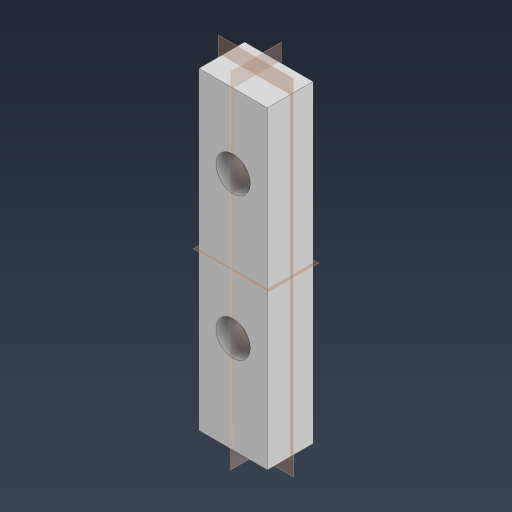
# Autodesk Inventor part: Направляющая
Saved by Autodesk Inventor 2023.2 (Build 272271030, 271C)
## iProperties
Created: 2026-01-04
Part Number: Направляющая
Material: Типовые
Document SubType Name: Modeling
Designer: Олег Коноваленко
Density: 1 g/cm^3
Appearance: По умолчанию
Author: Олег Коноваленко
Autodesk Inventor part; units mm, degrees
sketch "Эскиз1" plane through (0, 0, 0) normal (0, 1, 0) x (-1, 0, 0)
  line L0 (6, 4) -> (-6, 4)
  line L1 (-6, 4) -> (-6, -4)
  line L2 (-6, -4) -> (6, -4)
  line L3 (6, -4) -> (6, 4)
  line L4 (6, 4) -> (-6, -4) construction
  line L5 (-6, 4) -> (6, -4) construction
  point P0 (0, 0)
  dimension "d0" = 12
  dimension "d1" = 8
  constraints: 12 end point, 2 midpoint, 2 parallel, 1 horizontal, 1 perpendicular
  measures "d0" distance of L1.end L2.end
  measures "d1" distance of L0.end L1.end
extrude "Выдавливание1" add sketch "Эскиз1" along normal mid plane 55
sketch "Эскиз2" plane through (-6, 27.5, 4) normal (0, 0, 1) x (1, 0, 0)
  circle A0 centre (6, -13) radius 1.75
  line L0 (0, 0) -> (12, 0) projected
  line L1 (6, 11) -> (6, -66) construction
  point P0 (6, -27.5)
  dimension "d4" = 13
  dimension "d5" = 3.5
  constraints: 1 centre point, 1 point on line
  measures "d4" distance from line of L0 A0.centre
  measures "d5" diameter of A0
extrude "Выдавливание2" cut sketch "Эскиз2" against normal up to next
sketch "Эскиз3" plane through (-6, 27.5, 4) normal (0, 0, 1) x (1, 0, 0)
  circle A0 centre (6, -13) radius 1.75 projected
  circle A1 centre (6, -13) radius 3
  point P0 (6, -27.5)
  dimension "d8" = 6
  constraints: 1 centre point, 1 coincident
  measures "d8" diameter of A1
extrude "Выдавливание3" cut sketch "Эскиз3" against normal blind 4.5
pattern_linear "Прямоуг.массив1" count 2 spacing 25 along (0, -1, 0) of "Выдавливание3", "Выдавливание2"
